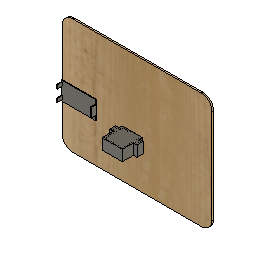
fire danger sign (Autodesk Fusion 360 design; units mm, degrees)
Autodesk Fusion 360 part; units mm, degrees
note: some values were not read from the file. Set by a fixed rule: which face or edge a step refers to.
sketch "Sketch1" plane through (0, 0, 0) normal (0, 0, 1) x (1, 0, 0) in component "Servo"
  line L0 (0, 0) -> (22.5, 0)
  line L1 (22.5, 0) -> (22.5, 15.7)
  line L2 (22.5, 15.7) -> (27.4, 15.7)
  line L3 (27.4, 15.7) -> (27.4, 18.2)
  line L4 (27.4, 18.2) -> (22.5, 18.2)
  line L5 (0, 0) -> (0, 15.7)
  line L6 (0, 15.7) -> (-4.9, 15.7)
  line L7 (-4.9, 15.7) -> (-4.9, 18.2)
  line L8 (-4.9, 18.2) -> (0, 18.2)
  line L9 (0, 18.2) -> (0, 22.4)
  line L10 (22.5, 18.2) -> (22.5, 26.7)
  line L11 (22.5, 26.7) -> (18.88, 26.7)
  line L12 (18.88, 26.7) -> (18.88, 29.7)
  line L13 (18.88, 29.7) -> (14.02, 29.7)
  line L14 (14.02, 29.7) -> (14.02, 26.7)
  line L15 (14.02, 26.7) -> (10.4, 26.7)
  line L16 (0, 22.4) -> (10.4, 22.4)
  line L17 (10.4, 22.4) -> (10.4, 26.7)
  dimension "d1" = 22.5
  dimension "d2" = 15.7
  dimension "d3" = 4.9
  dimension "d4" = 2.5
  dimension "d5" = 15.7
  dimension "d6" = 4.9
  dimension "d7" = 2.5
  dimension "d8" = 4.2
  dimension "d9" = 8.5
  dimension "d10" = 3.62
  dimension "d11" = 3
  dimension "d12" = 4.86
  dimension "d13" = 3.62
  constraint coincident L0.start L5.start
  constraint horizontal L0
  constraint perpendicular L0 L1
  constraint perpendicular L1 L2
  constraint perpendicular L0 L3
  constraint perpendicular L1 L4
  constraint perpendicular L0 L5
  constraint perpendicular L5 L6
  constraint perpendicular L0 L7
  constraint perpendicular L5 L8
  constraint perpendicular L6 L9
  constraint perpendicular L4 L10
  constraint perpendicular L10 L11
  constraint perpendicular L4 L12
  constraint perpendicular L10 L13
  constraint perpendicular L13 L14
  constraint perpendicular L14 L15
  constraint perpendicular L9 L16
  constraint perpendicular L15 L17
  measures "d1" distance of L0.start L0.end
  measures "d2" distance of L0.end L1.end
  measures "d3" distance of L1.end L2.end
  measures "d4" distance of L2.end L3.end
  measures "d5" distance of L0.start L5.end
  measures "d6" distance of L5.end L6.end
  measures "d7" distance of L6.end L7.end
  measures "d8" distance of L8.end L9.end
  measures "d9" distance of L4.end L10.end
  measures "d10" distance of L10.end L11.end
  measures "d11" distance of L11.end L12.end
  measures "d12" distance of L12.end L13.end
  measures "d13" distance of L14.end L15.end
extrude "Extrude1" add sketch "Sketch1" along normal blind 12.1 makes body 1 in component "Servo"
sketch "Sketch2" plane through (0, 26.7, 0) normal (0, 1, 0) x (-1, 0, 0) in component "Servo"
  line L0 (-22.5, 0) -> (-18.88, 0)
  line L1 (-18.88, 0) -> (-18.88, 12.1)
  line L2 (-18.88, 12.1) -> (-22.5, 12.1)
  line L3 (-22.5, 12.1) -> (-22.5, 0)
  circle A0 centre (-16.45, 6.05) radius 6.05
  circle A1 centre (-16.45, 6.05) radius 2.43
  line L4 (-18.88, 11.5905) -> (-18.88, 0.5095)
  line L5 (-14.02, 11.5905) -> (-14.02, 0.5095)
  line L6 (-22.5, 12.1) -> (-10.4, 12.1)
  line L7 (-10.4, 12.1) -> (-10.4, 0)
  line L8 (-10.4, 0) -> (-22.5, 0)
  line L9 (-22.5, 0) -> (-22.5, 12.1)
  line L10 (-18.88, 11.5905) -> (-18.88, 12.1)
  line L11 (-14.02, 11.5905) -> (-14.02, 12.1)
  line L12 (-14.02, 0.5095) -> (-14.02, 0)
  line L13 (-18.88, 0.5095) -> (-18.88, 0)
  dimension "d16" = 4.86
  dimension "d19" = 12.1
  dimension "d20" = 12.1
  constraint tangent L0 A0
  constraint tangent L3 A0
  constraint tangent L2 A0
  constraint coincident A0 L4.start
  constraint coincident L1 L4.start
  constraint coincident A0 L4.end
  constraint coincident L1 L4.end
  constraint coincident A0 L5.start
  constraint coincident A0 L5.end
  constraint parallel L1 L5
  constraint horizontal L6
  constraint vertical L7
  constraint horizontal L8
  constraint vertical L9
  constraint coincident L2.end L3.start
  constraint coincident L1.end L2.start
  constraint coincident L6 L11.end
  constraint perpendicular L6 L11
  constraint coincident L8 L12.end
  constraint perpendicular L8 L12
  constraint coincident L0.end L1.start
  measures "d16" diameter of A1
  measures "d19" distance of L2.end L6.end
  measures "d20" distance of L2.end L0.start
extrude "Extrude2" cut sketch "Sketch2" along normal blind 3 contours L1 A0 L8 L13 | L1 A0 A1 L4 L5 | A0 L8 L12 | L1 A0 A1 L4 L5 | L1 A0 L6 L10 | A0 L6 L11 bodies 1 in component "Servo"
extrude "Extrude3" cut sketch "Sketch2" against normal blind 4.3 contours L0 L1 L3 A0 L8 L9 L13 | L1 A0 L8 L13 | L1 L2 L3 A0 L6 L9 L10 | A0 L8 L12 | L1 A0 L6 L10 | A0 L7 L8 L12 | A0 L6 L11 | A0 L6 L7 L11 bodies 1 in component "Servo"
sketch "Sketch1 (2)" plane through (0, 29.7, 0) normal (0, 1, 0) x (-1, 0, 0) in component "Servo Horn"
  circle A0 centre (-16.45, 6.05) radius 2.43
  circle A1 centre (-16.45, 6.05) radius 3.375
  line L0 (-16.45, 6.05) -> (-0.45, 6.05) construction
  circle A2 centre (-0.45, 6.05) radius 2 construction
  line L1 (-16.16, 9.4125) -> (-0.2781, 8.0426)
  line L2 (-16.16, 2.6875) -> (-0.2781, 4.0574)
  arc A3 (-0.2781, 4.0574) -> (-0.2781, 8.0426) centre (-0.45, 6.05) ccw
  dimension "d23" = 6.75
  dimension "d37" = 16
  dimension "d38" = 4
  constraint concentric A0 A1
  constraint coincident A0.centre A1.centre
  constraint horizontal L0
  constraint coincident L0.end A2.centre
  constraint coincident A1 L1.start
  constraint coincident A2 L1.end
  constraint tangent A1 L1
  constraint tangent A2 L1
  constraint coincident A1 L2.start
  constraint coincident A2 L2.end
  constraint tangent A2 L2
  constraint tangent A1 L2
  measures "d23" diameter of A1
  measures "d37" distance of A0.centre L0.end
  measures "d38" diameter of A2
extrude "Extrude1'" add sketch "Sketch1 (2)" against normal blind 3 separate body contours A1 makes body 2 in component "Servo Horn"
extrude "Extrude2'" add sketch "Sketch1 (2)" along normal blind 1.25 bodies 2 in component "Servo Horn"
sketch "Sketch1 (3)" plane through (0, 26.7, 0) normal (0, 1, 0) x (-1, 0, 0) in component "Sign"
  circle A0 centre (-16.45, 6.05) radius 6.05
  circle A1 centre (-16.45, 6.05) radius 2.43
  line L0 (-16.45, 6.05) -> (-16.45, 0) construction
  line L1 (-16.45, 0) -> (-121.45, 0) construction
  circle A2 centre (-16.45, 6.05) radius 4.43
  line L2 (-121.45, 0) -> (-121.45, -54) construction
  line L3 (-121.45, -54) -> (88.55, -54) construction
  line L4 (88.55, -54) -> (88.55, 108) construction
  line L5 (88.55, 108) -> (-121.45, 108) construction
  line L6 (-121.45, 108) -> (-121.45, 0) construction
  circle A3 centre (-106.45, 93) radius 15 construction
  circle A4 centre (73.55, 93) radius 15 construction
  circle A5 centre (73.55, -39) radius 15 construction
  circle A6 centre (-106.45, -39) radius 15 construction
  arc A7 (-121.45, -39) -> (-106.45, -54) centre (-106.45, -39) ccw
  arc A8 (73.55, -54) -> (88.55, -39) centre (73.55, -39) ccw
  arc A9 (88.55, 93) -> (73.55, 108) centre (73.55, 93) ccw
  arc A10 (-106.45, 108) -> (-121.45, 93) centre (-106.45, 93) ccw
  line L7 (-106.45, 108) -> (73.55, 108)
  line L8 (88.55, 93) -> (88.55, -39)
  line L9 (73.55, -54) -> (-106.45, -54)
  line L10 (-121.45, -39) -> (-121.45, 93)
  point P0 (-16.45, 6.05)
  dimension "d39" = 105
  dimension "d41" = 2
  dimension "d42" = 54
  dimension "d43" = 210
  dimension "d44" = 162
  dimension "d45" = 15
  dimension "d46" = 15
  dimension "d47" = 15
  dimension "d48" = 15
  constraint coincident P0 A0.centre
  constraint coincident A0 L0.end
  constraint vertical L0
  constraint tangent A0 L1
  constraint perpendicular L1 L2
  constraint perpendicular L2 L3
  constraint perpendicular L3 L4
  constraint perpendicular L2 L5
  constraint perpendicular L1 L6
  constraint tangent L6 A3
  constraint tangent L5 A3
  constraint tangent L5 A4
  constraint tangent L4 A4
  constraint tangent L3 A5
  constraint tangent L4 A5
  constraint tangent L3 A6
  constraint tangent L2 A6
  constraint coincident L2 A7.start
  constraint coincident A6 A7.end
  constraint coincident A6.centre A7.centre
  constraint coincident L4 A8.end
  constraint coincident L3 A8.start
  constraint coincident A5 A8.start
  constraint coincident L4 A9.start
  constraint coincident L5 A9.end
  constraint coincident A4 A9.end
  constraint coincident A3 A10.start
  constraint coincident A3 A10.end
  constraint coincident A3.centre A10.centre
  constraint tangent A9 L7
  constraint tangent A6 L9
  constraint tangent A3 L10
  measures "d39" distance of L0.end L1.end
  measures "d42" distance of L1.end L2.end
  measures "d43" distance of L2.end L3.end
  measures "d44" distance of L3.end L4.end
  measures "d45" radius of A3
  measures "d46" radius of A4
  measures "d47" radius of A5
  measures "d48" radius of A6
extrude "Extrude1''" add sketch "Sketch1 (3)" along normal blind 2.2 separate body contours A0 | A7 A8 A9 A10 L7 L8 L9 L10 makes body 3 in component "Sign"
sketch "Sketch1 (4)" plane through (0, 0, 0) normal (0, 0, -1) x (1, 0, 0) in component "Servo Mount"
  line L0 (0, -22.4) -> (16.45, -22.4)
  line L1 (16.45, -22.4) -> (22.5, -22.4)
  line L2 (22.5, -22.4) -> (22.5, -18.2)
  line L3 (22.5, -18.2) -> (27.4, -18.2)
  line L4 (27.4, -18.2) -> (27.4, -15.7)
  line L5 (27.4, -15.7) -> (22.5, -15.7)
  line L6 (22.5, -15.7) -> (22.5, 0)
  line L7 (22.5, 0) -> (0, 0)
  line L8 (0, 0) -> (0, -15.7)
  line L9 (0, -15.7) -> (-4.9, -15.7)
  line L10 (-4.9, -15.7) -> (-4.9, -18.2)
  line L11 (-4.9, -18.2) -> (0, -18.2)
  line L12 (0, -18.2) -> (0, -22.4)
  line L13 (-1.5, -14.2) -> (-6.4, -14.2)
  line L14 (-6.4, -14.2) -> (-6.4, -19.7)
  line L15 (-6.4, -19.7) -> (-1.5, -19.7)
  line L16 (-1.5, -19.7) -> (-1.5, -23.9)
  line L17 (-1.5, -23.9) -> (16.45, -23.9)
  line L18 (16.45, -23.9) -> (24, -23.9)
  line L19 (24, -23.9) -> (24, -19.7)
  line L20 (24, -19.7) -> (28.9, -19.7)
  line L21 (28.9, -19.7) -> (28.9, -14.2)
  line L22 (28.9, -14.2) -> (24, -14.2)
  line L23 (24, -14.2) -> (24, 1.5)
  line L24 (24, 1.5) -> (-1.5, 1.5)
  line L25 (-1.5, 1.5) -> (-1.5, -14.2)
  line L26 (-0.5, -15.2) -> (-5.4, -15.2)
  line L27 (-5.4, -15.2) -> (-5.4, -18.7)
  line L28 (-5.4, -18.7) -> (-0.5, -18.7)
  line L29 (-0.5, -18.7) -> (-0.5, -22.9)
  line L30 (-0.5, -22.9) -> (16.45, -22.9)
  line L31 (16.45, -22.9) -> (23, -22.9)
  line L32 (23, -22.9) -> (23, -18.7)
  line L33 (23, -18.7) -> (27.9, -18.7)
  line L34 (27.9, -18.7) -> (27.9, -15.2)
  line L35 (27.9, -15.2) -> (23, -15.2)
  line L36 (23, -15.2) -> (23, 0.5)
  line L37 (23, 0.5) -> (-0.5, 0.5)
  line L38 (-0.5, 0.5) -> (-0.5, -15.2)
  dimension "d51" = 1.5
  dimension "d52" = 0.5
extrude "Extrude1'''" add sketch "Sketch1 (4)" against normal blind 13.1 separate body contours L13 L14 L15 L16 L17 L18 L19 L20 L21 L22 L23 L24 L25 makes body 4 in component "Servo Mount"
extrude "Extrude2''" add sketch "Sketch1 (4)" 1 faces at (7.3333, -1.1667, 0) along normal blind 1 contours L0 L1 L2 L3 L4 L5 L6 L7 L8 L9 L10 L11 L12 | L26 L27 L28 L29 L30 L31 L32 L33 L34 L35 L36 L37 L38 on bodies 4 bodies 4 in component "Servo Mount"
sketch "Sketch2 (2)" plane through (-0.5, 0, 0) normal (1, 0, 0) x (0, 1, 0) in component "Servo Mount"
  line L0 (-0.5, 0) -> (15.2, 0)
  line L1 (15.2, 0) -> (15.2, 13.1)
  line L2 (15.2, 13.1) -> (-0.5, 13.1)
  line L3 (-0.5, 13.1) -> (-0.5, 0)
  circle A0 centre (2.6108, 6.55) radius 3.1108
  constraint tangent L3 A0
extrude "Extrude3'" cut sketch "Sketch2 (2)" against normal blind 1 contours A0 bodies 4 in component "Servo Mount"
sketch "Sketch3" plane through (0, 0, 13.1) normal (0, 0, 1) x (-1, 0, 0) in component "Servo Mount"
  line L0 (0.5, 0.5) -> (0.5, -15.2)
  line L1 (0.5, -15.2) -> (5.4, -15.2)
  line L2 (5.4, -15.2) -> (5.4, -18.7)
  line L3 (5.4, -18.7) -> (0.5, -18.7)
  line L4 (0.5, -18.7) -> (0.5, -22.9)
  line L5 (0.5, -22.9) -> (-23, -22.9)
  line L6 (-23, -22.9) -> (-23, -18.7)
  line L7 (-23, -18.7) -> (-27.9, -18.7)
  line L8 (-27.9, -18.7) -> (-27.9, -15.2)
  line L9 (-27.9, -15.2) -> (-23, -15.2)
  line L10 (-23, -15.2) -> (-23, 0.5)
  line L11 (-23, 0.5) -> (0.5, 0.5)
  line L12 (1.5, -14.2) -> (1.5, 1.5)
  line L13 (1.5, 1.5) -> (-24, 1.5)
  line L14 (-24, 1.5) -> (-24, -14.2)
  line L15 (-24, -14.2) -> (-28.9, -14.2)
  line L16 (-28.9, -14.2) -> (-28.9, -19.7)
  line L17 (-28.9, -19.7) -> (-24, -19.7)
  line L18 (-24, -19.7) -> (-24, -23.9)
  line L19 (-24, -23.9) -> (1.5, -23.9)
  line L20 (1.5, -23.9) -> (1.5, -19.7)
  line L21 (1.5, -19.7) -> (6.4, -19.7)
  line L22 (6.4, -19.7) -> (6.4, -14.2)
  line L23 (6.4, -14.2) -> (1.5, -14.2)
  line L24 (6.9, -20.2) -> (6.9, -13.7)
  line L25 (6.9, -13.7) -> (2, -13.7)
  line L26 (2, -13.7) -> (2, 2)
  line L27 (2, 2) -> (-24.5, 2)
  line L28 (-24.5, 2) -> (-24.5, -13.7)
  line L29 (-24.5, -13.7) -> (-29.4, -13.7)
  line L30 (-29.4, -13.7) -> (-29.4, -20.2)
  line L31 (-29.4, -20.2) -> (-24.5, -20.2)
  line L32 (-24.5, -20.2) -> (-24.5, -24.4)
  line L33 (-24.5, -24.4) -> (2, -24.4)
  line L34 (2, -24.4) -> (2, -20.2)
  line L35 (2, -20.2) -> (6.9, -20.2)
  line L36 (7.9, -21.2) -> (7.9, -12.7)
  line L37 (7.9, -12.7) -> (3, -12.7)
  line L38 (3, -12.7) -> (3, 3)
  line L39 (3, 3) -> (-25.5, 3)
  line L40 (-25.5, 3) -> (-25.5, -12.7)
  line L41 (-25.5, -12.7) -> (-30.4, -12.7)
  line L42 (-30.4, -12.7) -> (-30.4, -21.2)
  line L43 (-30.4, -21.2) -> (-25.5, -21.2)
  line L44 (-25.5, -21.2) -> (-25.5, -25.4)
  line L45 (-25.5, -25.4) -> (3, -25.4)
  line L46 (3, -25.4) -> (3, -21.2)
  line L47 (3, -21.2) -> (7.9, -21.2)
  dimension "d59" = 0.5
  dimension "d60" = 1.5
extrude "Extrude4" add sketch "Sketch3" along normal blind 1 separate body contours L0 L1 L2 L3 L4 L5 L6 L7 L8 L9 L10 L11 | L12 L13 L14 L15 L16 L17 L18 L19 L20 L21 L22 L23 | L24 L25 L26 L27 L28 L29 L30 L31 L32 L33 L34 L35 | L36 L37 L38 L39 L40 L41 L42 L43 L44 L45 L46 L47 makes body 5 in component "Servo Mount"
extrude "Extrude5" add sketch "Sketch3" against normal blind 14.1 contours L36 L37 L38 L39 L40 L41 L42 L43 L44 L45 L46 L47 bodies 5 in component "Servo Mount"
sketch "Sketch4" plane through (-2, 0, 0) normal (1, 0, 0) x (0, 1, 0) in component "Servo Mount"
  line L0 (13.7, 13.1) -> (-2, 13.1)
  line L1 (-2, 13.1) -> (-2, -1)
  line L2 (-2, -1) -> (13.7, -1)
  line L3 (13.7, -1) -> (13.7, 13.1)
  circle A0 centre (2.6689, 6.5488) radius 3.1059
extrude "Extrude6" cut sketch "Sketch4" against normal blind 1 contours A0 bodies 5 in component "Servo Mount"
sketch "Sketch5" plane through (0, 22.9, 0) normal (0, -1, 0) x (1, 0, 0) in component "Servo Mount"
  line L0 (-0.5, 0) -> (23, 0)
  line L1 (23, 0) -> (23, 13.1)
  line L2 (23, 13.1) -> (-0.5, 13.1)
  line L3 (-0.5, 13.1) -> (-0.5, 0)
  line L4 (23, 13.1) -> (9, 13.1)
  line L5 (9, 13.1) -> (9, 0)
  line L6 (9, 0) -> (23, 0)
  line L7 (23, 0) -> (23, 13.1)
  dimension "d67" = 14
  constraint horizontal L4
  constraint vertical L5
  constraint horizontal L6
  constraint vertical L7
  constraint coincident L0 L5.end
  constraint coincident L1.end L2.start
  measures "d67" distance of L1.end L4.end
extrude "Extrude4'" cut sketch "Sketch5" against normal blind 2.5 contours L0 L1 L2 L4 L5 L6 L7 bodies 1 makes body 6 at (14.0336, 25.4, 6.9699) in component "Servo"
extrude "Extrude7" cut sketch "Sketch5" against normal blind 2.5 contours L0 L1 L2 L4 L5 L6 L7 bodies 4 5 in component "Servo Mount"
sketch "Sketch1 (5)" plane through (0, 26.7, 0) normal (0, -1, 0) x (1, 0, 0) in component "ESP32 Mount"
  circle A0 centre (16.45, 6.05) radius 4.43
  arc A1 (-88.55, -39) -> (-73.55, -54) centre (-73.55, -39) ccw
  line L0 (-73.55, -54) -> (106.45, -54)
  arc A2 (106.45, -54) -> (121.45, -39) centre (106.45, -39) ccw
  line L1 (121.45, -39) -> (121.45, 93)
  arc A3 (121.45, 93) -> (106.45, 108) centre (106.45, 93) ccw
  line L2 (106.45, 108) -> (-73.55, 108)
  arc A4 (-73.55, 108) -> (-88.55, 93) centre (-73.55, 93) ccw
  line L3 (-88.55, 93) -> (-88.55, -39)
  line L4 (-88.55, 27) -> (-87.55, 27) construction
  line L5 (-87.55, 27) -> (-42.55, 27) construction
  line L6 (-42.55, 27) -> (-42.55, 1.5) construction
  line L7 (-42.55, 1.5) -> (-87.55, 1.5) construction
  line L8 (-87.55, 1.5) -> (-87.55, 27) construction
  line L9 (-87.55, 27) -> (-87.55, 25) construction
  line L10 (-87.55, 1.5) -> (-87.55, 3.5) construction
  line L11 (-87.55, 3.5) -> (-88.55, 3.5)
  line L12 (-88.55, 3.5) -> (-88.55, 8.5)
  line L13 (-88.55, 8.5) -> (-87.55, 8.5)
  line L14 (-87.55, 8.5) -> (-87.55, 3.5)
  line L15 (-87.55, 25) -> (-88.55, 25)
  line L16 (-88.55, 25) -> (-88.55, 20)
  line L17 (-88.55, 20) -> (-87.55, 20)
  line L18 (-87.55, 20) -> (-87.55, 25)
  line L19 (-42.55, 14.25) -> (-41.55, 14.25) construction
  line L20 (-41.55, 14.25) -> (-41.55, 20.625) construction
  line L21 (-41.55, 20.625) -> (-40.55, 20.625)
  line L22 (-40.55, 20.625) -> (-40.55, 7.875)
  line L23 (-40.55, 7.875) -> (-41.55, 7.875)
  line L24 (-41.55, 7.875) -> (-41.55, 20.625)
  line L25 (-88.55, 25) -> (-88.55, 27)
  line L26 (-88.55, 27) -> (-40.55, 27)
  line L27 (-40.55, 27) -> (-40.55, 20.625)
  line L28 (-40.55, 7.875) -> (-40.55, 1.5)
  line L29 (-40.55, 1.5) -> (-88.55, 1.5)
  line L30 (-88.55, 3.5) -> (-88.55, 1.5)
  line L31 (-88.55, 8.5) -> (-88.55, 20)
  dimension "d72" = 1
  dimension "d73" = 45
  dimension "d74" = 25.5
  dimension "d75" = 2
  dimension "d76" = 2
  dimension "d77" = 5
  dimension "d78" = 5
  dimension "d79" = 1
  dimension "d80" = 6.375
  dimension "d81" = 1
  dimension "d82" = 12.75
  constraint midpoint L3 L4.start
  constraint horizontal L4
  constraint horizontal L5
  constraint vertical L6
  constraint horizontal L7
  constraint vertical L8
  constraint coincident L8 L9.end
  constraint perpendicular L7 L10
  constraint horizontal L11
  constraint vertical L12
  constraint horizontal L13
  constraint vertical L14
  constraint coincident L3 L12.end
  constraint horizontal L15
  constraint vertical L16
  constraint horizontal L17
  constraint vertical L18
  constraint coincident L3 L16.end
  constraint midpoint L6 L19.start
  constraint perpendicular L6 L19
  constraint perpendicular L19 L20
  constraint horizontal L21
  constraint vertical L22
  constraint horizontal L23
  constraint vertical L24
  constraint perpendicular L22 L26
  constraint perpendicular L21 L27
  constraint perpendicular L7 L28
  constraint coincident L3 L29.end
  constraint perpendicular L3 L29
  constraint perpendicular L29 L30
  measures "d72" distance of L4.start L4.end
  measures "d73" distance of L4.end L5.end
  measures "d74" distance of L4.end L7.end
  measures "d75" distance of L4.end L9.end
  measures "d76" distance of L7.end L10.end
  measures "d77" distance of L10.end L13.end
  measures "d78" distance of L9.end L17.end
  measures "d79" distance of L19.start L19.end
  measures "d80" distance of L19.end L20.end
  measures "d81" distance of L20.end L21.end
  measures "d82" distance of L20.end L23.end
extrude "Extrude1''''" add sketch "Sketch1 (5)" along normal blind 1 separate body contours L3 L11 L13 L14 L15 L17 L18 L21 L23 L24 L25 L26 L27 L28 L29 L30 L31 makes body 7 in component "ESP32 Mount"
extrude "Extrude2'''" add sketch "Sketch1 (5)" along normal blind 7 contours L3 L11 L12 L13 L14 | L3 L15 L16 L17 L18 bodies 7 in component "ESP32 Mount"
extrude "Extrude6'" add sketch "Sketch1 (5)" along normal blind 5.5 contours L21 L22 L23 L24 bodies 7 in component "ESP32 Mount"
extrude "Extrude3''" add 4 faces at (-88.2167, 19.7, 23.3333) (-88.2167, 19.7, 6.8333) (-88.2167, 19.7, 6.8333) (-88.2167, 19.7, 23.3333) along direction (0, -1, 0) blind 1 separate body on bodies 7 makes body 8 at (-87.55, 19.3667, 6.8333) makes body 9 at (-88.55, 19.3667, 23.3333) in component "ESP32 Mount"
extrude "Extrude7'" add 1 faces at (-40.8833, 21.2, 12.125) along direction (0, -1, 0) blind 1 separate body on bodies 7 makes body 10 in component "ESP32 Mount"
extrude "Extrude4''" add 2 faces at (-87.55, 19.3667, 21.6667) (-87.55, 19.3667, 6.8333) along direction (1, 0, 0) blind 1 on bodies 8 9 bodies 7 10 9 8 in component "ESP32 Mount"
extrude "Extrude5'" add 1 faces at (-41.55, 20.8667, 12.125) along direction (-1, 0, 0) blind 1 on bodies 10 bodies 7 10 in component "ESP32 Mount"
chamfer "Chamfer1" distance 1 angle 45 3 edges at (-42.55, 21.2, 14.25) (-86.55, 19.7, 22.5) (-86.55, 19.7, 6) on bodies 7 in component "ESP32 Mount"
sketch "Sketch1 (6)" plane through (0, 30.95, 0) normal (0, 1, 0) x (-1, 0, 0) in component "Arrow"
  circle A0 centre (-16.45, 6.05) radius 2.43
  arc A1 (-16.16, 9.4125) -> (-16.16, 2.6875) centre (-16.45, 6.05) ccw
  line L0 (-16.16, 2.6875) -> (-0.2781, 4.0574)
  arc A2 (-0.2781, 4.0574) -> (-0.2781, 8.0426) centre (-0.45, 6.05) ccw
  line L1 (-0.2781, 8.0426) -> (-16.16, 9.4125)
  circle A3 centre (-16.45, 6.05) radius 3.3625 construction
  line L2 (-13.0875, 2.6875) -> (-13.0875, 9.4125) construction
  line L3 (-13.0875, 9.4125) -> (-19.8125, 9.4125) construction
  line L4 (-19.8125, 9.4125) -> (-19.8125, 2.6875) construction
  line L5 (-19.8125, 2.6875) -> (-13.0875, 2.6875) construction
  line L6 (-19.8125, 9.4125) -> (30.1875, 9.4125)
  line L7 (30.1875, 9.4125) -> (30.1875, 2.6875) construction
  line L8 (30.1875, 2.6875) -> (-19.8125, 2.6875)
  line L9 (-19.8125, 2.6875) -> (-19.8125, 9.4125)
  line L10 (30.1875, 9.4125) -> (30.1875, 2.6875) construction
  line L11 (30.1875, 2.6875) -> (36.0115, 6.05)
  line L12 (36.0115, 6.05) -> (30.1875, 9.4125)
  point P0 (-16.45, 6.05)
  point P1 (32.1288, 6.05)
  dimension "d94" = 50
  dimension "d95" = 6.725
  constraint concentric A0 A3
  constraint coincident P0 A0.centre
  constraint horizontal L6
  constraint vertical L7
  constraint horizontal L8
  constraint vertical L9
  measures "d94" distance of L3.end L6.end
  measures "d95" distance of L3.end L4.end
extrude "Extrude1'''''" [rolled back] along distance 2 taper angle -20 in component "Arrow"
component "Servo" placed x (1, 0, 0) y (0, 1, 0) z (0, 0, 1) at (0, 0, 0)
component "Servo Horn" placed x (1, 0, 0) y (0, 1, 0) z (0, 0, 1) at (0, 0, 0)
component "Sign" placed x (1, 0, 0) y (0, 1, 0) z (0, 0, 1) at (0, 0, 0)
component "Servo Mount" placed x (1, 0, 0) y (0, 1, 0) z (0, 0, 1) at (0, 0, 0)
component "ESP32 Mount" placed x (1, 0, 0) y (0, 1, 0) z (0, 0, 1) at (0, 0, 0)
named bodies: "Bottom", "Top"
